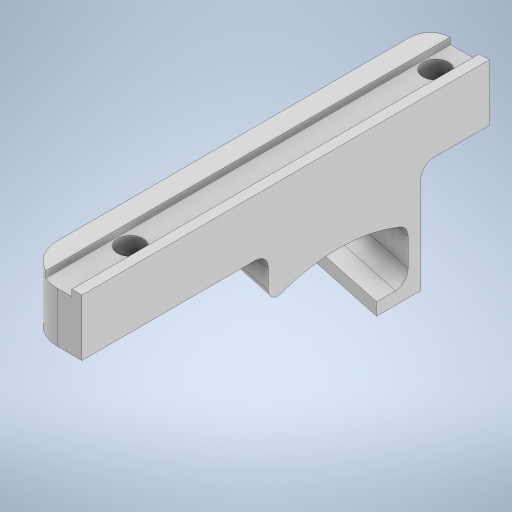
# Autodesk Inventor part: Right-Brush-Top
Saved by Autodesk Inventor 2024 (Build 280153000, 153)
## iProperties
Created: 2023-12-13
Part Number: Right-Brush-Top
Material: Generic
Document SubType Name: Modeling
Designer: shaun
Density: 1 g/cm^3
Appearance: Default
Author: shaun
Autodesk Inventor part; units mm, degrees
ref_plane "YZ Plane" through (0, 0, 0) normal (1, 0, 0) x (0, 1, 0)
ref_plane "XZ Plane" through (0, 0, 0) normal (0, 1, 0) x (-1, 0, 0)
ref_plane "XY Plane" through (0, 0, 0) normal (0, 0, 1) x (1, 0, 0)
sketch "Sketch1" plane through (0, 0, 0) normal (0, 1, 0) x (-1, 0, 0)
  line L0 (0, 64.7) -> (11, 64.7) construction
  line L1 (11, 64.7) -> (11, 0) construction
  line L2 (11, 0) -> (0, 0) construction
  line L3 (0, 0) -> (0, 64.7) construction
  line L4 (5.5, 64.7) -> (5.5, 0) construction
  line L5 (11, 32.35) -> (0, 32.35) construction
  circle A0 centre (5.5, 53.1) radius 1.6 construction
  circle A1 centre (5.5, 53.1) radius 2.05
  circle A2 centre (5.5, 43.4) radius 1.6 construction
  circle A3 centre (5.5, 43.4) radius 2.05 construction
  circle A4 centre (5.5, 33.7) radius 1.6 construction
  circle A5 centre (5.5, 33.7) radius 2.05 construction
  circle A6 centre (5.5, 24) radius 1.6 construction
  circle A7 centre (5.5, 24) radius 2.05 construction
  circle A8 centre (5.5, 14.3) radius 1.6 construction
  circle A9 centre (5.5, 14.3) radius 2.05 construction
  circle A10 centre (5.5, 4.6) radius 1.6 construction
  circle A11 centre (5.5, 4.6) radius 2.05
  line L6 (7.8, 64.7) -> (3.2, 64.7) construction
  line L7 (3.2, 64.7) -> (3.2, 0)
  line L8 (3.2, 0) -> (7.8, 0) construction
  line L9 (7.8, 0) -> (7.8, 64.7)
  circle A12 centre (5.5, 53.1) radius 2.3 construction
  circle A13 centre (5.5, 59.2) radius 5.5 construction
  circle A14 centre (7.8, 3.2) radius 3.2 construction
  line L10 (0, 0) -> (3.2, 0) construction
  line L11 (1.6, 0) -> (1.6, 64.7)
  circle A15 centre (5.5, 4.6) radius 3.5
  circle A16 centre (5.5, 14.3) radius 3.5 construction
  circle A17 centre (5.5, 24) radius 3.5 construction
  circle A18 centre (5.5, 33.7) radius 3.5 construction
  circle A19 centre (5.5, 43.4) radius 3.5 construction
  circle A20 centre (5.5, 53.1) radius 3.5
  arc A21 (7.8, 0) -> (11, 3.2) centre (7.8, 3.2) ccw
  arc A22 (11, 59.2) -> (5.5, 64.7) centre (5.5, 59.2) ccw
  line L12 (11, 3.2) -> (11, 59.2)
  line L13 (1.6, 0) -> (7.8, 0)
  line L14 (1.6, 64.7) -> (5.5, 64.7)
  point P0 (5.5, 54.7)
  point P1 (5.5, 3)
  point P2 (-5.6396, 32.0975)
  point P3 (-5.6396, -32.6025)
  point P4 (-1.0396, 31.5935)
  point P5 (7.8, 64.196)
  point P6 (7.8, 55.7382)
  point P7 (7.8, 50.4618)
  point P8 (3.2, 0)
  point P9 (3.2, 50.4618)
  point P10 (3.2, 55.7382)
  dimension "d4" = 3.2
  dimension "d5" = 4.1
  dimension "d6" = 9.7
  dimension "d7" = 6.5
  dimension "d8" = 10
  dimension "d9" = 3
  dimension "d10" = 0.7
  dimension "d11" = 3.2
  dimension "d12" = 7
  constraints: 30 end point, 21 centre point, 17 coincident, 10 point on line, 8 point on circle, 5 equal radius, 5 midpoint, 5 parallel, 5 tangent, 3 perpendicular, 2 collinear, 2 horizontal, 2 line through centre, 2 vertical, 2 vertical alignment, 22 other
  measures "d5" diameter of A1
  measures "d6" distance of point (5.5, 53.1) A2.centre
  measures "d8" distance from line of L0 point (5.5, 54.7)
  measures "d9" distance of L4.end point (5.5, 3)
  measures "d11" distance between parallel lines of L1 L9
  measures "d12" diameter of A15
extrude "Extrusion1" add sketch "Sketch1" along normal blind 6 contours L7 A20 A15 L13 L11 L14 | L7 A20 | A20 L9 | L9 A22 L12 A21 A15 A20 | L7 A15 | A15 L9
extrude "Extrusion2" add sketch "Sketch1" along normal blind 5 contours L14 A22 L9 A20 L7 | A20 L9 L7 | A20 L9 A15 L7 | A15 L9 L7 | L7 A15 L9 L13
extrude "Extrusion3" add sketch "Sketch1" against normal blind 3 contours L14 A22 L9 A20 L7 | L7 A20 A15 L13 L11 L14 | A20 L9 A15 L7 | L9 A22 L12 A21 A15 A20 | L7 A15 L9 L13
sketch "Sketch2" plane through (0, -3, 0) normal (0, -1, 0) x (1, 0, 0)
  line L0 (-5.5, 53.1) -> (-5.5, 4.6) construction
  circle A0 centre (-5.5, 53.1) radius 4.85 construction
  circle A1 centre (-5.5, 43.4) radius 4.85 construction
  circle A2 centre (-5.5, 33.7) radius 4.85 construction
  circle A3 centre (-5.5, 24) radius 4.85 construction
  circle A4 centre (-5.5, 14.3) radius 4.85 construction
  circle A5 centre (-5.5, 4.6) radius 4.85 construction
  line L1 (-11, 3.2) -> (-11, 59.2) construction
  line L2 (0, 35.1) -> (-11, 35.1) construction
  line L3 (-11, 35.1) -> (-11, 12.9) construction
  line L4 (-11, 12.9) -> (0, 12.9) construction
  line L5 (0, 12.9) -> (0, 35.1) construction
  line L6 (0, 35.1) -> (-11, 12.9) construction
  line L7 (-11, 35.1) -> (0, 12.9) construction
  point P0 (0, 0)
  dimension "d20" = 22.2
  constraints: 14 end point, 10 equal radius, 7 coincident, 6 centre point, 5 point on line, 2 midpoint, 2 parallel, 1 horizontal, 1 perpendicular, 1 vertical
  measures "d20" distance between parallel lines of L4 L2
ref_plane "Work Plane1" through (-11, -3, 12.9) normal (0, 0, -1) x (-1, 0, 0)
sketch "Sketch3" plane through (-11, -3, 12.9) normal (0, 0, -1) x (-1, 0, 0)
  line L0 (0, 0) -> (-9.4, 0)
  line L1 (0, 0) -> (9.4, 0) construction
  line L2 (9.4, 0) -> (9.4, -2.4) construction
  line L3 (0, 0) -> (0, -14.7868)
  line L4 (0, -14.7868) -> (-9.4, -17.3055)
  line L5 (-9.4, -17.3055) -> (-9.4, 0)
  line L6 (-9.4, -15.3055) -> (0, -12.7868)
  line L7 (9.4, -2.4) -> (0, -4.9187) construction
  line L8 (0, -4.9187) -> (-9.4, -7.4374)
  line L9 (9.4, -2.4) -> (0, -2.4) construction
  line L10 (0, -12.7868) -> (-1.967, -5.4458) construction
  point P0 (-11, 3)
  dimension "d32" = 2.4
  dimension "d34" = 15
  dimension "d35" = 7.6
  dimension "d36" = 2
  constraints: 22 end point, 6 point on line, 3 parallel, 3 perpendicular, 2 collinear, 2 horizontal, 1 vertical
  measures "d32" distance of L2.end L1.end
  measures "d34" angle of L9 L7
  measures "d35" distance of L6.end L10.end
  measures "d36" distance of L3.end L6.end
extrude "Extrusion4" add sketch "Sketch3" along normal blind 2
extrude "Extrusion5" add sketch "Sketch3" against normal blind 22.2 contours L3 L8 L5 L0
extrude "Extrusion6" add sketch "Sketch3" against normal blind 5 contours L3 L4 L5 L6
ref_plane "Work Plane3" through (-9.033, -8.4458, 12.9) normal (-0.9659258, 0.258819, 0) x (-0.258819, -0.9659258, 0)
sketch "Sketch5" plane through (-9.033, -8.4458, 12.9) normal (-0.9659258, 0.258819, 0) x (-0.258819, -0.9659258, 0)
  line L0 (0, 0) -> (0, 22.2) projected
  arc A0 (0, 22.2) -> (0, 0) centre (24.4688, 11.1) ccw
  point P0 (-10.4959, -12.9)
  point P1 (-2.4, 11.1)
  point P2 (0, 11.1)
  dimension "d37" = 2.4
  constraints: 3 point on circle, 1 centre point, 1 midpoint
  measures "d37" distance of point (-2.4, 11.1) point (0, 11.1)
extrude "Extrusion7" cut sketch "Sketch5" along normal through all both and the other way through all
fillet "Fillet1" radius 2 4 edges at (-6.3, -3, 10.9) (-6.3, -3, 35.1) (-6.3, -9.1781, 12.9) (-6.3, -17.0462, 12.9)
fillet "Fillet2" radius 1.5 1 edges at (-6.3, -9.1781, 35.1)
body "Solid1"
